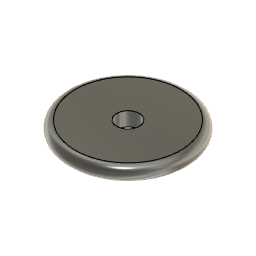
wheel right rear (Autodesk Fusion 360 design; units mm, degrees)
Autodesk Fusion 360 part; units mm, degrees
mesh "Mesh1" [no effect] in component "wheel right rear"
sketch "top" plane through (0, 0, 0) normal (0, 0, 1) x (1, 0, 0) in component "wheel right rear"
  circle A0 centre (0, 0) radius 3.2
  circle A1 centre (0, 0) radius 15
  circle A2 centre (0, 0) radius 17
  dimension "d182_1" = 34
  constraint concentric A0 A1
  constraint concentric A0 A2
  measures "d182_1" diameter of A2
sketch "side" plane through (0, 0, 0) normal (0, 1, 0) x (1, 0, 0) in component "wheel right rear"
  line L0 (-15, 0) -> (-15, -4)
  constraint vertical L0
extrude "Extrude1" add sketch "top" along normal blind 4 contours A1 | A2 in component "wheel right rear"
fillet "Fillet1" radius 2 2 edges at (-15.8496, -6.1475, 4) (-15.8496, -6.1475, 0) in component "wheel right rear"
component "wheel right rear" placed x (1, 0, 0) y (0, 1, 0) z (0, 0, 1) at (0, 0, 0)
named bodies: "wheel right rear"
